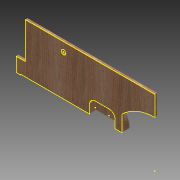
# Autodesk Inventor part: Shooter_TopMotorSupportRight
Saved by Autodesk Inventor 2014 (Build 180170000, 170)
## iProperties
Created: 2016-01-27
Part Number: Shooter_TopMotorSupportRight
Material: Generic
Document SubType Name: Modeling
Designer: Ian
Density: 1 g/cm^3
Appearance: Birch - Natural Polished
Author: Ian
Autodesk Inventor part; units mm, degrees
ref_plane "YZ Plane" through (0, 0, 0) normal (1, 0, 0) x (0, 1, 0)
ref_plane "XZ Plane" through (0, 0, 0) normal (0, 1, 0) x (-1, 0, 0)
ref_plane "XY Plane" through (0, 0, 0) normal (0, 0, 1) x (1, 0, 0)
sketch "Sketch1" plane through (0, 0, 0) normal (0, 0, 1) x (1, 0, 0)
  circle A0 centre (0, 0) radius 12.7
  arc A1 (50.8, 0) -> (-50.8, 0) centre (0, 0) ccw
  line L0 (-50.8, 0) -> (-50.8, -225.3234)
  line L1 (-50.8, -225.3234) -> (50.8, -225.3234)
  line L2 (50.8, -225.3234) -> (50.8, 0)
  circle A2 centre (176.5046, -179.1208) radius 32.385
  circle A3 centre (253.9746, -179.1208) radius 32.385
  line L3 (144.1196, -225.3234) -> (144.1196, -179.1208)
  line L4 (286.3596, -225.3234) -> (286.3596, -179.1208)
  line L5 (176.5046, -146.7358) -> (253.9746, -146.7358)
  line L6 (50.8, -225.3234) -> (144.1196, -225.3234)
  line L7 (286.3596, -225.3234) -> (508, -225.3234)
  line L8 (-50.8, -225.3234) -> (-238.2266, -225.3234)
  line L9 (-263.6266, -225.3234) -> (-263.6266, -150.876)
  line L10 (-263.6266, -150.876) -> (-212.8266, -150.876)
  line L11 (-212.8266, -150.876) -> (-212.8266, 50.8)
  line L12 (-212.8266, 50.8) -> (508, 50.8)
  line L13 (508, 50.8) -> (508, -225.3234)
  line L14 (-238.2266, -229.108) -> (-238.2266, -225.3234)
  line L15 (-238.2266, -229.108) -> (-263.6266, -229.108)
  line L16 (-263.6266, -229.108) -> (-263.6266, -225.3234)
  dimension "d0" = 176.5046
  dimension "d1" = 179.1208
  dimension "d2" = 64.77
  dimension "d3" = 64.77
  dimension "d4" = 77.47
  dimension "d5" = 212.8266
  dimension "d6" = 50.8
  dimension "d7" = 150.876
  dimension "d8" = 508
  dimension "d9" = 229.108
  constraints: 34 end point, 8 perpendicular, 6 point on circle, 4 centre point, 3 parallel, 2 tangent, 1 coincident, 1 collinear
  measures "d0" horizontal distance of point (176.505, -179.121) A0.centre
  measures "d1" vertical distance of A0.centre point (176.505, -179.121)
  measures "d2" diameter of A2
  measures "d3" diameter of A3
  measures "d4" distance of point (176.505, -179.121) A3.centre
  measures "d5" distance of L0.end L9.start
  measures "d6" distance of L9.end L10.end
  measures "d7" distance from line of A0.centre L10
  measures "d8" distance from line of L13 A0.centre
  measures "d9" vertical distance of L14.start A1.centre
extrude "Extrusion1" add sketch "Sketch1" along normal blind 12.7 contours L2 L1 L0 A1 | A1 L12 L13 L7 L4 A3 L5 A2 L3 L6 L2 | A1 L0 L8 L14 L15 L16 L9 L10 L11 L12
sketch "Sketch2" plane through (0, 0, 0) normal (0, 0, -1) x (-1, 0, 0)
  line L0 (-286.3596, -225.3234) -> (-324.4596, -225.3234)
  line L1 (-324.4596, -225.3234) -> (-324.4596, -136.4234)
  line L2 (-324.4596, -136.4234) -> (-286.3596, -136.4234)
  line L3 (-286.3596, -136.4234) -> (-286.3596, -225.3234)
  line L4 (-144.1196, -225.3234) -> (-106.0196, -225.3234)
  line L5 (-106.0196, -225.3234) -> (-106.0196, -136.4234)
  line L6 (-106.0196, -136.4234) -> (-144.1196, -136.4234)
  line L7 (-144.1196, -136.4234) -> (-144.1196, -225.3234)
  dimension "d12" = 38.1
  dimension "d13" = 88.9
  dimension "d14" = 38.1
  dimension "d15" = 88.9
  constraints: 16 end point, 4 parallel, 2 horizontal, 2 perpendicular
  measures "d12" distance of L1.end L2.end
  measures "d13" distance of L0.end L1.end
  measures "d14" distance of L6.end L5.end
  measures "d15" distance of L5.end L4.end
extrude "Extrusion2" add sketch "Sketch2" along normal blind 25.4
sketch "Sketch3" plane through (0, 0, -25.4) normal (0, 0, -1) x (-1, 0, 0)
  line L0 (-324.4596, -136.4234) -> (-106.0196, -136.4234)
  line L1 (-106.0196, -136.4234) -> (-106.0196, -225.3234)
  line L2 (-106.0196, -225.3234) -> (-324.4596, -225.3234)
  line L3 (-324.4596, -225.3234) -> (-324.4596, -136.4234)
  line L4 (-106.0196, -136.4234) -> (-106.0196, -225.3234) projected
  circle A0 centre (-225.1964, -177.5746) radius 12.7
  circle A1 centre (0, 0) radius 12.7 projected
  dimension "d18" = 88.9
  dimension "d19" = 0
  dimension "d20" = 25.4
  dimension "d21" = 225.1964
  constraints: 8 end point, 2 parallel, 1 centre point, 1 horizontal, 1 perpendicular
  measures "d18" distance of L0.end L1.end
  measures "d19" distance between parallel lines of L4 L1
  measures "d20" diameter of A0
  measures "d21" horizontal distance of A0.centre A1.centre
extrude "Extrusion3" add sketch "Sketch3" along normal blind 12.7 contours L0 L1 L2 L3
sketch "Sketch4" plane through (0, 0, 12.7) normal (0, 0, 1) x (1, 0, 0)
  line L0 (286.3596, -225.3234) -> (508, -225.3234) projected
  line L1 (324.4596, -136.4234) -> (508, -60.2234)
  line L2 (508, -60.2234) -> (366.7969, -60.2234)
  arc A0 (508, -60.2234) -> (324.4596, -136.4234) centre (508, -319.3672) ccw
  line L3 (324.4596, -136.4234) -> (324.4596, -225.3234)
  line L4 (508, -60.2234) -> (324.4596, -60.2234)
  line L5 (324.4596, -60.2234) -> (324.4596, -225.3234)
  line L6 (324.4596, -225.3234) -> (508, -225.3234)
  line L7 (508, -225.3234) -> (508, -60.2234)
  constraints: 14 end point, 2 parallel, 2 perpendicular, 2 point on circle, 1 centre point, 1 horizontal, 1 point on line, 1 tangent
extrude "Extrusion4" cut sketch "Sketch4" against normal blind 25.4 contours L3 L1 L7 L0 | A0 L1
sketch "Sketch5" plane through (0, 0, -38.1) normal (0, 0, -1) x (-1, 0, 0)
  line L0 (-324.4596, -136.4234) -> (-324.4596, -225.3234) projected
  line L1 (-106.0196, -225.3234) -> (-106.0196, -136.4234) projected
  line L2 (-106.0196, -136.4234) -> (-324.4596, -136.4234) projected
  arc A0 (-235.5596, -136.4234) -> (-324.4596, -225.3234) centre (-235.5596, -225.3234) ccw
  line L3 (-324.4596, -225.3234) -> (-235.5596, -136.4234) construction
  line L4 (-324.4596, -225.3234) -> (-198.736, -225.3234) construction
  arc A1 (-106.0196, -225.3234) -> (-194.9196, -136.4234) centre (-194.9196, -225.3234) ccw
  line L5 (-106.0196, -225.3234) -> (-194.9196, -136.4234) construction
  line L6 (-106.0196, -225.3234) -> (19.704, -225.3234) construction
  point P0 (0, 0)
  dimension "d26" = 45
  dimension "d27" = 135
  constraints: 8 end point, 4 point on circle, 4 tangent, 2 centre point, 2 equal length, 2 horizontal, 2 point on line
  measures "d26" angle of L4 L3
  measures "d27" angle of L6 L5
extrude "Extrusion5" cut sketch "Sketch5" against normal blind 38.1
fillet "Fillet1" radius 12.7 3 edges at (215.2396, -136.4234, -38.1) (132.0578, -162.4616, -38.1) (298.4214, -162.4616, -38.1)
sketch "Sketch6" plane through (0, 0, 12.7) normal (0, 0, 1) x (1, 0, 0)
  arc A0 (508, -60.2234) -> (324.4596, -136.4234) centre (508, -319.3672) ccw projected
  line L0 (508, -60.2234) -> (508, 50.8) projected
  line L1 (508, 50.8) -> (-212.8266, 50.8) projected
  line L2 (-212.8266, 50.8) -> (-212.8266, -150.876) projected
  line L3 (-212.8266, -150.876) -> (-263.6266, -150.876) projected
  line L4 (-263.6266, -150.876) -> (-263.6266, -229.108) projected
  line L5 (-263.6266, -229.108) -> (-238.2266, -229.108) projected
  line L6 (-238.2266, -229.108) -> (-238.2266, -225.3234) projected
  line L7 (-238.2266, -225.3234) -> (144.1196, -225.3234) projected
  line L8 (144.1196, -225.3234) -> (144.1196, -179.1208) projected
  arc A1 (176.5046, -146.7358) -> (144.1196, -179.1208) centre (176.5046, -179.1208) ccw projected
  line L9 (176.5046, -146.7358) -> (253.9746, -146.7358) projected
  arc A2 (286.3596, -179.1208) -> (253.9746, -146.7358) centre (253.9746, -179.1208) ccw projected
  line L10 (286.3596, -179.1208) -> (286.3596, -225.3234) projected
  line L11 (286.3596, -225.3234) -> (324.4596, -225.3234) projected
  line L12 (324.4596, -225.3234) -> (324.4596, -136.4234) projected
  circle A3 centre (0, 0) radius 12.7 projected
sketch "Sketch7" plane through (0, 0, 12.7) normal (0, 0, 1) x (1, 0, 0)
  line L0 (324.4596, -225.3234) -> (324.4596, -136.4234) projected
  circle A0 centre (0, 0) radius 12.7 projected
  line L1 (12.7, 0) -> (283.972, 0)
  circle A1 centre (283.972, 0) radius 35.56
  dimension "d31" = 271.272
  dimension "d32" = 71.12
  constraints: 2 end point, 1 centre point, 1 coincident, 1 horizontal alignment, 1 perpendicular, 1 other
  measures "d31" distance of L1.start L1.end
  measures "d32" diameter of A1
extrude "Extrusion6" cut sketch "Sketch7" against normal blind 25.4 contours A1
body "Solid1"
